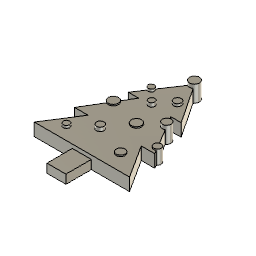
christmastree (Autodesk Fusion 360 design; units mm, degrees)
part number: 2025-10-29-14-43-43-000
Autodesk Fusion 360 part; units mm, degrees
sketch "Sketch1" plane through (0, 0, 0) normal (0, 0, 1) x (1, 0, 0)
  line L0 (0, 0) -> (15, 0)
  line L1 (15, 0) -> (15, 20)
  line L2 (15, 20) -> (0, 20)
  line L3 (0, 20) -> (0, 0)
  line L4 (0, 20) -> (-30, 20)
  line L5 (15, 20) -> (45, 20)
  line L6 (45, 20) -> (28.4651, 45.8146)
  line L7 (28.4651, 45.8146) -> (39.0949, 45.8146)
  line L8 (39.0949, 45.8146) -> (20.1808, 77.3096)
  line L9 (20.1808, 77.3096) -> (28.3002, 77.3096)
  line L10 (28.3002, 77.3096) -> (7.5, 108.6082)
  line L11 (-13.3002, 77.3096) -> (7.5, 108.6082)
  line L12 (-5.1808, 77.3096) -> (-13.3002, 77.3096)
  line L13 (-24.0949, 45.8146) -> (-5.1808, 77.3096)
  line L14 (-13.4651, 45.8146) -> (-24.0949, 45.8146)
  line L15 (-30, 20) -> (-13.4651, 45.8146)
  dimension "d1" = 15
  dimension "d2" = 20
  dimension "d3" = 30
  constraint horizontal L0
  constraint vertical L1
  constraint horizontal L2
  constraint vertical L3
  constraint coincident L0.start L3.end
  constraint perpendicular L3 L4
  constraint perpendicular L1 L5
  constraint parallel L5 L7
  constraint parallel L7 L9
  measures "d1" distance of L0.start L0.end
  measures "d2" distance of L0.start L2.end
  measures "d3" distance of L1.end L5.end
extrude "Extrude1" add sketch "Sketch1" along normal blind 10 contours L2 L4 L5 L6 L7 L8 L9 L10 L11 L12 L13 L14 L15
extrude "Extrude2" add sketch "Sketch1" along normal blind 7 contours L0 L1 L2 L3
sketch "Sketch2" plane through (0, 0, 10) normal (0, 0, 1) x (-1, 0, 0)
  line L0 (30, -20) -> (-45, -20)
  line L1 (-45, -20) -> (-28.4651, -45.8146)
  line L2 (-28.4651, -45.8146) -> (-39.0949, -45.8146)
  line L3 (-39.0949, -45.8146) -> (-20.1808, -77.3096)
  line L4 (-20.1808, -77.3096) -> (-28.3002, -77.3096)
  line L5 (-28.3002, -77.3096) -> (-7.5, -108.6082)
  line L6 (-7.5, -108.6082) -> (13.3002, -77.3096)
  line L7 (13.3002, -77.3096) -> (5.1808, -77.3096)
  line L8 (5.1808, -77.3096) -> (24.0949, -45.8146)
  line L9 (24.0949, -45.8146) -> (13.4651, -45.8146)
  line L10 (13.4651, -45.8146) -> (30, -20)
  circle A0 centre (6.0624, -88.2005) radius 2.5
  circle A1 centre (-24.9742, -69.3278) radius 3.5
  circle A2 centre (-0.4251, -41.565) radius 3
  circle A3 centre (-25.1078, -32.9073) radius 3.5
  circle A4 centre (-13.8678, -88.9006) radius 3
  circle A5 centre (12.6203, -64.9216) radius 4
  circle A6 centre (-4.4215, -78.0323) radius 2.5
  circle A7 centre (-11.665, -58.7996) radius 4
  circle A8 centre (-7.5, -108.6082) radius 4
  circle A9 centre (14.6379, -30.0753) radius 2.5
  circle A10 centre (-35.8887, -51.1535) radius 3
  dimension "d8" = 5
  dimension "d9" = 7
  dimension "d10" = 6
  dimension "d11" = 7
  dimension "d12" = 6
  dimension "d13" = 8
  dimension "d14" = 5
  dimension "d15" = 8
  dimension "d16" = 8
  dimension "d17" = 5
  dimension "d18" = 6
  constraint coincident L6 A0.centre
  constraint coincident L3 A1.centre
  constraint coincident L8 A5.centre
  constraint coincident L5.end L6.start
  constraint coincident L3 A10.centre
  measures "d8" diameter of A0
  measures "d9" diameter of A1
  measures "d10" diameter of A2
  measures "d11" diameter of A3
  measures "d12" diameter of A4
  measures "d13" diameter of A5
  measures "d14" diameter of A6
  measures "d15" diameter of A7
  measures "d16" diameter of A8
  measures "d17" diameter of A9
  measures "d18" diameter of A10
extrude "Extrude3" add sketch "Sketch2" along normal blind 3 contours L3 A1 | L3 A1 | L5 L6 A8 | L5 L6 A8 | A2 | A6
extrude "Extrude4" add sketch "Sketch2" along normal blind 2 contours L6 A0 | L6 A0 | A4 | A9
extrude "Extrude5" add sketch "Sketch2" along normal blind 1 contours L8 A5 | L8 A5 | L3 A10 | L3 A10 | A3 | A7
extrude "Extrude6" add sketch "Sketch2" against normal blind 10 contours L8 A5 | L3 A10 | L3 A1 | L6 A0 | L5 L6 A8 picked at (13.8963, -64.5349) picked at (-37.2683, -51.7586) picked at (-26.1307, -69.1738) picked at (6.8875, -88.0837) picked at (-4.8478, -108.804)
sketch "Sketch3" plane through (0, 0, 0) normal (0, 0, 1) x (1, 0, 0)
  line L0 (45, 20) -> (15, 20)
  line L1 (15, 20) -> (15, 0)
  line L2 (15, 0) -> (0, 0)
  line L3 (0, 0) -> (0, 20)
  line L4 (0, 20) -> (-30, 20)
  line L5 (-30, 20) -> (-13.4651, 45.8146)
  line L6 (-13.4651, 45.8146) -> (-24.0949, 45.8146)
  line L7 (-24.0949, 45.8146) -> (-14.6797, 61.4925)
  arc A0 (-10.561, 68.3508) -> (-14.6797, 61.4925) centre (-12.6203, 64.9216) ccw
  line L8 (-10.561, 68.3508) -> (-5.1808, 77.3096)
  line L9 (-5.1808, 77.3096) -> (-13.3002, 77.3096)
  line L10 (-13.3002, 77.3096) -> (-7.4461, 86.1184)
  arc A1 (-4.6787, 90.2827) -> (-7.4461, 86.1184) centre (-6.0624, 88.2005) ccw
  line L11 (-4.6787, 90.2827) -> (5.286, 105.2768)
  arc A2 (9.714, 105.2768) -> (5.286, 105.2768) centre (7.5, 108.6082) ccw
  line L12 (9.714, 105.2768) -> (28.3002, 77.3096)
  line L13 (28.3002, 77.3096) -> (20.1808, 77.3096)
  line L14 (20.1808, 77.3096) -> (23.1723, 72.3283)
  arc A3 (26.7762, 66.3273) -> (23.1723, 72.3283) centre (24.9742, 69.3278) ccw
  line L15 (26.7762, 66.3273) -> (34.3442, 53.7254)
  arc A4 (37.4332, 48.5817) -> (34.3442, 53.7254) centre (35.8887, 51.1535) ccw
  line L16 (37.4332, 48.5817) -> (39.0949, 45.8146)
  line L17 (39.0949, 45.8146) -> (28.4651, 45.8146)
  line L18 (28.4651, 45.8146) -> (45, 20)
  circle A5 centre (4.4215, 78.0323) radius 2.5
  circle A6 centre (-12.6203, 64.9216) radius 4
  line L19 (7.5, 108.6082) -> (-13.3002, 77.3096)
  circle A7 centre (-6.0624, 88.2005) radius 2.5
  circle A8 centre (13.8678, 88.9006) radius 3
  circle A9 centre (7.5, 108.6082) radius 4
  circle A10 centre (24.9742, 69.3278) radius 3.5
  circle A11 centre (24.9742, 69.3278) radius 3.5
  circle A12 centre (11.665, 58.7996) radius 4
  circle A13 centre (0.4251, 41.565) radius 3
  circle A14 centre (25.1078, 32.9073) radius 3.5
  circle A15 centre (-14.6379, 30.0753) radius 2.5
  circle A16 centre (35.8887, 51.1535) radius 3
  line L20 (0, 20) -> (0, 0)
  line L21 (0, 0) -> (15, 0)
  line L22 (15, 0) -> (15, 20)
  line L23 (15, 20) -> (0, 20)
